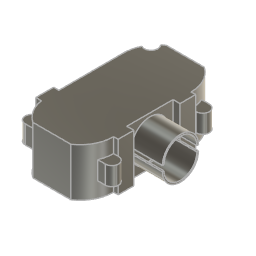
nerfaccel v3 (Autodesk Fusion 360 design; units mm, degrees)
Autodesk Fusion 360 part; units mm, degrees
sketch "Sketch1" plane through (0, 0, 0) normal (0, 0, 1) x (1, 0, 0)
  line L0 (0, 0) -> (38.8, 0)
  line L1 (38.8, 0) -> (38.8, -76.6)
  line L2 (38.8, -76.6) -> (0, -76.6)
  line L3 (0, -76.6) -> (0, 0)
  circle A0 centre (19.4, -60.5516) radius 19.4
  line L4 (0, -38.3) -> (38.8, -38.3)
  circle A1 centre (19.4, -16.0484) radius 19.4
  point P0 (8.5, -76.6)
  point P1 (30.3, -76.6)
  dimension "d1" = 38.8
  dimension "d2" = 76.6
  dimension "d3" = 21.8
  constraint horizontal L0
  constraint vertical L1
  constraint horizontal L2
  constraint vertical L3
  constraint coincident L0.start L3.end
  constraint tangent L1 A0
  constraint tangent L3 A0
  constraint coincident A0 P0
  constraint coincident L2 P0
  constraint coincident L2 P1
  constraint coincident A0 P1
  constraint midpoint L3 L4.start
  constraint midpoint L1 L4.end
  constraint symmetric A0 L4 A1
  measures "d1" distance of L0.start L0.end
  measures "d2" distance of L0.start L2.end
  measures "d3" distance of P0 P1
extrude "Extrude1" add sketch "Sketch1" along normal blind 27.6 contours L0 A1 | L1 L3 L4 A1 | L1 L3 A0 L4 | L2 A0 picked at (18.9167, -11.798) picked at (21.2355, -62.094)
ref_plane "WorkPlane1" through (19.4, -38.3, 13.8) normal (0, 0, 1) x (1, 0, 0)
sketch "Sketch3" plane through (0, 0, 13.8) normal (0, 0, 1) x (1, 0, 0)
  line L0 (38.8, -60.5516) -> (38.8, -16.0484)
  arc A0 (38.8, -16.0484) -> (30.3, 0) centre (19.4, -16.0484) ccw
  line L1 (30.3, 0) -> (8.5, 0)
  arc A1 (8.5, 0) -> (0, -16.0484) centre (19.4, -16.0484) ccw
  line L2 (0, -16.0484) -> (0, -60.5516)
  arc A2 (30.3, -76.6) -> (38.8, -60.5516) centre (19.4, -60.5516) ccw
  line L3 (8.5, -76.6) -> (30.3, -76.6)
  arc A3 (0, -60.5516) -> (8.5, -76.6) centre (19.4, -60.5516) ccw
  line L4 (38.8, -16.0484) -> (45.4494, -16.0484)
  line L5 (45.4494, -16.0484) -> (45.4494, -8.4484)
  line L6 (45.4494, -8.4484) -> (37.2494, -8.4484)
  circle A4 centre (41.6494, -12.2484) radius 3.8
  line L7 (41.4, -16.0484) -> (41.4, -25.0484)
  line L8 (41.4, -25.0484) -> (38.8, -25.0484)
  line L9 (38.8, -38.3) -> (0, -38.3)
  line L10 (41.4, -51.5516) -> (38.8, -51.5516)
  line L11 (41.4, -60.5516) -> (41.4, -51.5516)
  circle A5 centre (41.6494, -64.3516) radius 3.8
  line L12 (45.4494, -60.5516) -> (45.4494, -68.1516)
  line L13 (45.4494, -68.1516) -> (37.2494, -68.1516)
  line L14 (38.8, -60.5516) -> (45.4494, -60.5516)
  line L15 (0, -26.8) -> (0, -49.8)
  line L16 (0, -53.2) -> (-3, -53.2)
  line L17 (-3, -53.2) -> (-3, -63.4)
  line L18 (-3, -63.4) -> (0.2102, -63.4)
  line L19 (-3, -63.4) -> (-5.2816, -63.4)
  line L20 (-5.2816, -63.4) -> (-5.2816, -71.1)
  line L21 (-5.2816, -71.1) -> (3.1184, -71.1)
  circle A6 centre (-1.4316, -67.25) radius 3.85
  circle A7 centre (3.9, -4.1484) radius 3.9
  line L22 (0, -4.1484) -> (0, -16.0484)
  dimension "d12" = 7.6
  dimension "d13" = 8.2
  dimension "d14" = 9
  dimension "d15" = 2.6
  dimension "d22" = 3.4
  dimension "d23" = 23
  dimension "d24" = 10.2
  dimension "d25" = 3
  dimension "d26" = 7.7
  dimension "d27" = 8.4
  dimension "d28" = 7.8
  dimension "d29" = 11.9
  constraint coincident L0.end A0.start
  constraint perpendicular L0 L4
  constraint perpendicular L4 L5
  constraint coincident A0 L6.end
  constraint perpendicular L5 L6
  constraint tangent L4 A4
  constraint tangent L5 A4
  constraint tangent L6 A4
  constraint coincident L4 L7.start
  constraint perpendicular L4 L7
  constraint coincident L0 L8.end
  constraint perpendicular L0 L8
  constraint midpoint L0 L9.start
  constraint midpoint L2 L9.end
  constraint symmetric L0.end L9 L0.start
  constraint symmetric L4.end L9 L12.start
  constraint symmetric L5.end L9 L12.end
  constraint symmetric L6.end L9 L13.end
  constraint symmetric A4 L9 A5
  constraint symmetric L7.start L9 L11.start
  constraint symmetric L7.end L9 L10.start
  constraint symmetric L8.end L9 L10.end
  constraint vertical L15
  constraint midpoint L2 L15
  constraint coincident L2 L16.start
  constraint perpendicular L2 L16
  constraint perpendicular L16 L17
  constraint perpendicular L2 L18
  constraint coincident A3 L18.end
  constraint perpendicular L17 L19
  constraint perpendicular L19 L20
  constraint tangent L19 A6
  constraint tangent L20 A6
  constraint tangent L21 A6
  constraint horizontal L21
  constraint coincident A3 L21.end
  constraint coincident A7 L22.start
  constraint tangent A7 L22
  constraint coincident A1.end L2.start
  constraint vertical L22
  measures "d12" distance of L4.end L5.end
  measures "d13" distance of L5.end L6.end
  measures "d14" distance of L7.start L7.end
  measures "d15" distance of L7.end L8.end
  measures "d22" distance of L15.end L16.start
  measures "d23" distance of L15.start L15.end
  measures "d24" distance of L16.end L17.end
  measures "d25" distance of L16.start L16.end
  measures "d26" distance of L19.end L20.end
  measures "d27" distance of L20.end L21.end
  measures "d28" diameter of A7
  measures "d29" distance of L22.start A1.end
extrude "Extrude4" add sketch "Sketch3" along normal mid plane 27.6 contours L0 L10 L11 L14 | L0 L4 L7 L8 | L2 A3 L16 L17 L18
extrude "Extrude5" cut 1 faces at (38.8, -42.7172, 9.2) along direction (-1, 0, 0) blind 1.4
sketch "Sketch2" plane through (37.4, 0, 0) normal (1, 0, 0) x (0, 1, 0)
  line L0 (-51.5516, 0) -> (-25.0484, 0)
  line L1 (-25.0484, 27.6) -> (-51.5516, 27.6)
  arc A0 (-27.95, 15.35) -> (-48.65, 15.35) centre (-38.3, 15.35) ccw
  arc A1 (-28.85, 15.35) -> (-47.75, 15.35) centre (-38.3, 15.35) ccw
  line L2 (-48.65, 15.35) -> (-47.75, 15.35)
  line L3 (-28.85, 15.35) -> (-27.95, 15.35)
  line L4 (-47.75, 15.35) -> (-28.85, 15.35)
  line L5 (-38.3, 27.6) -> (-38.3, 0)
  line L6 (-38.3, 13.8) -> (-30.0917, 13.8)
  arc A2 (-47.75, 12.25) -> (-28.85, 12.25) centre (-38.3, 12.25) ccw
  arc A3 (-48.65, 12.25) -> (-27.95, 12.25) centre (-38.3, 12.25) ccw
  line L7 (-28.85, 12.25) -> (-27.95, 12.25)
  line L8 (-48.65, 12.25) -> (-47.75, 12.25)
  line L9 (-51.5516, 27.6) -> (-51.5516, 0)
  line L10 (-25.0484, 0) -> (-25.0484, 27.6)
  line L11 (-51.5516, 27.6) -> (-51.5516, 0)
  line L12 (-51.5516, 0) -> (-25.0484, 0)
  line L13 (-25.0484, 0) -> (-25.0484, 27.6)
  line L14 (-25.0484, 27.6) -> (-51.5516, 27.6)
  point P0 (-38.3, 13.8)
  dimension "d6" = 10.35
  dimension "d7" = 0.9
  dimension "d8" = 1.55
  constraint coincident A0.centre A1.centre
  constraint horizontal L2
  constraint horizontal L3
  constraint horizontal L4
  constraint midpoint L1 L5.start
  constraint midpoint L0 L5.end
  constraint coincident A0.centre L5
  constraint coincident A0.centre L4
  constraint midpoint L5 P0
  constraint coincident P0 L6.start
  constraint perpendicular L5 L6
  constraint symmetric A0.start L6 A3.end
  constraint symmetric A0.end L6 A3.start
  constraint symmetric A0 L6 A3
  constraint symmetric A1.start L6 A2.end
  constraint symmetric A1.end L6 A2.start
  constraint symmetric A1 L6 A2
  measures "d6" radius of A0
  measures "d7" distance of A0 A1
  measures "d8" distance of A0.centre P0
extrude "Extrude2" add sketch "Sketch2" along normal blind 17.5 contours L5 A2 A3 L8 | L5 A2 A3 L7 | A0 A1 L2 L5 | A0 A1 L3 L5
extrude "Extrude6" add sketch "Sketch3" against normal blind 5.1 contours A2 A5 L14 | A2 A5 | A2 A5 L13 | A0 L4 A4 | A0 A4 | A1 A7 L22 | A0 L6 A4 | A1 A7 | A3 L21 A6 | A3 L18 A6 | A3 A6 picked at (40.8119, -64.1747) picked at (40.8119, -12.4253) picked at (2.9177, -3.4995) picked at (-1.0737, -67.1005)
extrude "Extrude7" add sketch "Sketch3" along normal blind 5.4 contours A2 A5 L14 | A2 A5 | A2 A5 L13 | A0 L4 A4 | A0 A4 | A1 A7 L22 | A0 L6 A4 | A1 A7 | A3 L21 A6 | A3 L18 A6 | A3 A6 picked at (40.8119, -64.1747) picked at (40.8119, -12.4253) picked at (2.9177, -3.4995) picked at (-1.0737, -67.1005)
sketch "Sketch4" plane through (0, 0, 0) normal (-1, 0, 0) x (0, -1, 0)
  line L0 (53.2, 0) -> (53.2, 27.6)
  line L1 (53.2, 27.6) -> (16.0484, 27.6)
  line L2 (16.0484, 27.6) -> (16.0484, 19.2)
  line L3 (16.0484, 19.2) -> (4.1484, 19.2)
  line L4 (4.1484, 19.2) -> (4.1484, 8.7)
  line L5 (4.1484, 8.7) -> (16.0484, 8.7)
  line L6 (16.0484, 8.7) -> (16.0484, 0)
  line L7 (16.0484, 0) -> (53.2, 0)
  line L8 (16.0484, 27.6) -> (63.4, 27.6)
  circle A0 centre (38.3, 13.8) radius 10
  point P0 (63.4, 27.6)
  point P1 (38.3, 13.8)
  dimension "d34" = 20
  constraint coincident L1.end L2.start
  constraint perpendicular L0 L8
  constraint coincident P0 L8.end
  constraint coincident P1 A0.centre
  measures "d34" diameter of A0
extrude "Extrude8" cut sketch "Sketch4" against normal blind 37.4 contours A0
sketch "Sketch5" plane through (0, 0, 19.2) normal (0, 0, 1) x (-1, 0, 0)
  arc A0 (-6.6733, 1.4063) -> (0, 4.1484) centre (-3.9, 4.1484) ccw
  line L0 (0, 4.1484) -> (0, 16.0484)
  arc A1 (-6.6733, 1.4063) -> (0, 16.0484) centre (-19.4, 16.0484) ccw
  circle A2 centre (-3.9, 4.1484) radius 3.9
  constraint concentric A0 A2
extrude "Extrude9" cut sketch "Sketch5" along normal blind 8.4 contours A1 A2
sketch "Sketch6" plane through (0, 0, 8.7) normal (0, 0, -1) x (1, 0, 0)
  arc A0 (0, 4.1484) -> (6.6733, 1.4063) centre (3.9, 4.1484) ccw
  arc A1 (0, 16.0484) -> (6.6733, 1.4063) centre (19.4, 16.0484) ccw
  line L0 (0, 16.0484) -> (0, 4.1484)
  circle A2 centre (3.9, 4.1484) radius 3.9
  constraint concentric A0 A2
extrude "Extrude10" cut sketch "Sketch6" along normal blind 8.7 contours A1 A2
equation "d6 = 20.7 mm / 2"
equation "d8 = ( 3.1 / 2 ) * 1 mm"
equation "d11 = -27.60 mm / 2"
equation "d20 = 2.6 mm - 4 mm"
equation "d30 = -13.80 mm + 8.7 mm"
equation "d32 = 13.80 mm - 8.4 mm"
